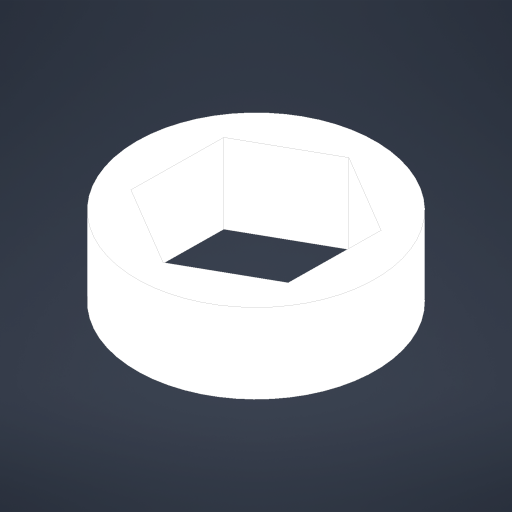
# Autodesk Inventor part: spacer
Saved by Autodesk Inventor 2024.3 (Build 283343000, 343)
## iProperties
Created: 2024-07-09
Part Number: spacer
Material: Generic
Document SubType Name: Modeling
Designer: kaito
Density: 1 g/cm^3
Appearance: Diamond plate - Dark Gray
Author: kaito
Autodesk Inventor part; units mm, degrees
ref_plane "YZ Plane" through (0, 0, 0) normal (1, 0, 0) x (0, 1, 0)
ref_plane "XZ Plane" through (0, 0, 0) normal (0, 1, 0) x (-1, 0, 0)
ref_plane "XY Plane" through (0, 0, 0) normal (0, 0, 1) x (1, 0, 0)
sketch "Sketch1" plane through (0, 0, 0) normal (0, 1, 0) x (-1, 0, 0)
  circle A0 centre (0, 0) radius 9.525
  line L0 (6.3918, 3.5928) -> (6.3073, -3.7391)
  line L1 (6.3073, -3.7391) -> (-0.0845, -7.3319)
  line L2 (-0.0845, -7.3319) -> (-6.3918, -3.5928)
  line L3 (-6.3918, -3.5928) -> (-6.3073, 3.7391)
  line L4 (-6.3073, 3.7391) -> (0.0845, 7.3319)
  line L5 (0.0845, 7.3319) -> (6.3918, 3.5928)
  point P0 (6.3496, -0.0731)
  dimension "d0" = 19.05
  dimension "d1" = 12.7
  constraints: 12 end point, 3 coincident, 1 centre point, 1 midpoint, 13 other
  measures "d0" diameter of A0
  measures "d1" distance from line of L3 point (6.35, -0.073)
extrude "Extrusion1" add sketch "Sketch1" along normal blind 6.35
body "Solid1"
